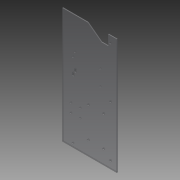
# Autodesk Inventor part: Electrical Board 2
Saved by Autodesk Inventor 2014 SP1 (Build 180222100, 222)
## iProperties
Created: 2013-12-13
Part Number: Electrical Board 2
Material: Polycarbonate, Clear
Document SubType Name: Modeling
Designer: Moses
Mass: 324.91 g
Surface Area: 1758.42 cm^2
Volume: 270.758 cm^3
Density: 1.2 g/cm^3
Appearance: Polycarbonate - Clear
Author: Moses
Autodesk Inventor part; units mm, degrees
ref_plane "YZ Plane" through (0, 0, 0) normal (1, 0, 0) x (0, 1, 0)
ref_plane "XZ Plane" through (0, 0, 0) normal (0, 1, 0) x (-1, 0, 0)
ref_plane "XY Plane" through (0, 0, 0) normal (0, 0, 1) x (1, 0, 0)
sketch "Sketch1" plane through (0, 0, 0) normal (0, 0, 1) x (1, 0, 0)
  line L0 (0, 0) -> (203.2, 0)
  line L1 (203.2, 0) -> (203.2, 431.8)
  line L2 (203.2, 431.8) -> (170.815, 431.8)
  line L3 (0, 431.8) -> (0, 0)
  circle A0 centre (177.8, 406.4) radius 3.3782
  circle A1 centre (177.8, 215.9) radius 3.3782
  circle A2 centre (177.8, 25.4) radius 3.3782
  line L4 (203.2, 215.9) -> (0, 215.9) construction
  line L5 (94.615, 431.8) -> (145.415, 393.7)
  line L6 (145.415, 393.7) -> (170.815, 393.7)
  line L7 (170.815, 393.7) -> (170.815, 431.8)
  line L8 (94.615, 431.8) -> (0, 431.8)
  line L9 (170.815, 431.8) -> (94.615, 431.8)
  circle A3 centre (139.7, 304.8) radius 2.3495
  line L10 (139.7, 304.8) -> (139.7, 246.634) construction
  circle A4 centre (139.7, 246.634) radius 2.3495
  circle A5 centre (45.6, 310.6) radius 2.54
  circle A6 centre (38.1, 292.1) radius 2.54
  line L11 (45.6, 310.6) -> (38.1, 310.6) construction
  line L12 (38.1, 310.6) -> (38.1, 292.1) construction
  line L13 (38.1, 292.1) -> (45.6, 292.1) construction
  line L14 (45.6, 292.1) -> (45.6, 310.6) construction
  circle A7 centre (38.1, 12.7) radius 2.3495
  line L15 (71.1544, 389.1684) -> (109.2544, 389.1684) construction
  line L16 (109.2544, 389.1684) -> (109.2544, 370.1184) construction
  line L17 (109.2544, 370.1184) -> (71.1544, 370.1184) construction
  line L18 (71.1544, 370.1184) -> (71.1544, 389.1684) construction
  line L19 (95.25, 165.1) -> (152.4, 165.1) construction
  line L20 (152.4, 165.1) -> (152.4, 50.8) construction
  line L21 (152.4, 50.8) -> (95.25, 50.8) construction
  line L22 (95.25, 50.8) -> (95.25, 165.1) construction
  circle A8 centre (95.25, 165.1) radius 3.175
  circle A9 centre (152.4, 165.1) radius 3.175
  circle A10 centre (152.4, 50.8) radius 3.175
  circle A11 centre (95.25, 50.8) radius 3.175
  line L23 (30.6, 229.55) -> (30.6, 259.55) projected
  arc A12 (30.6, 229.55) -> (34.6, 225.55) centre (34.6, 229.55) ccw projected
  line L24 (52.6, 225.55) -> (34.6, 225.55) projected
  line L25 (52.6, 225.55) -> (52.6, 263.55) projected
  line L26 (34.6, 263.55) -> (52.6, 263.55) projected
  arc A13 (34.6, 263.55) -> (30.6, 259.55) centre (34.6, 259.55) ccw projected
  arc A14 (49.81, 256.2) -> (44.31, 256.2) centre (47.06, 256.2) ccw projected
  line L27 (49.81, 256.2) -> (49.81, 248.7) projected
  arc A15 (44.31, 248.7) -> (49.81, 248.7) centre (47.06, 248.7) ccw projected
  line L28 (44.31, 248.7) -> (44.31, 256.2) projected
  arc A16 (41.85, 240.2) -> (36.35, 240.2) centre (39.1, 240.2) ccw projected
  line L29 (41.85, 240.2) -> (41.85, 232.7) projected
  arc A17 (36.35, 232.7) -> (41.85, 232.7) centre (39.1, 232.7) ccw projected
  line L30 (36.35, 232.7) -> (36.35, 240.2) projected
  circle A18 centre (30.4488, 139.597) radius 2.3812 projected
  circle A19 centre (64.8012, 139.597) radius 2.3812 projected
  circle A20 centre (30.4488, 106.323) radius 2.3812 projected
  circle A21 centre (64.8012, 106.323) radius 2.3812 projected
  dimension "d0" = 6.7564
  dimension "d3" = 190.5
  dimension "d8" = 25.4
  dimension "d9" = 431.8
  dimension "d10" = 203.2
  dimension "d14" = 38.1
  dimension "d15" = 76.2
  dimension "d16" = 25.4
  dimension "d17" = 4.699
  dimension "d18" = 58.166
  dimension "d19" = 63.5
  dimension "d20" = 127
  dimension "d26" = 5.08
  dimension "d27" = 18.5
  dimension "d28" = 7.5
  dimension "d29" = 38.1
  dimension "d30" = 76.2
  dimension "d31" = 4.699
  dimension "d32" = 38.1
  dimension "d33" = 12.7
  dimension "d34" = 32.385
  dimension "d35" = 19.05
  dimension "d36" = 38.1
  dimension "d37" = 57.15
  dimension "d38" = 6.35
  dimension "d39" = 114.3
  dimension "d40" = 50.8
  dimension "d41" = 50.8
  constraints: 46 end point, 12 centre point, 10 parallel, 5 coincident, 5 equal radius, 5 horizontal, 4 perpendicular, 3 vertical, 2 midpoint, 1 point on line, 4 other
  measures "d0" diameter of A0
  measures "d3" distance of A0.centre A1.centre
  measures "d8" distance from line of L1 A0.centre
  measures "d9" distance of L3.start L0.start
  measures "d10" distance of L0.start L0.end
  measures "d14" distance of L6.end L2.end
  measures "d15" distance of L2.end L5.start
  measures "d16" distance of L5.end L6.end
  measures "d17" diameter of A3
  measures "d18" distance of L10.start L10.end
  measures "d19" distance between parallel lines of L1 L10
  measures "d20" distance from line of L9 L10.start
  measures "d26" diameter of A5
  measures "d27" distance of L14.start L14.end
  measures "d28" distance of L12.end L14.start
  measures "d29" distance between parallel lines of L3 L12
  measures "d30" distance between parallel lines of L4 L13
  measures "d31" diameter of A7
  measures "d32" distance from line of A7.centre L3
  measures "d33" distance from line of L0 A7.centre
  measures "d34" distance between parallel lines of L1 L7
  measures "d35" distance of L15.end L16.end
  measures "d36" distance of L16.end L17.end
  measures "d37" distance of L19.start L19.end
  measures "d38" diameter of A8
  measures "d39" distance of L21.end L19.start
  measures "d40" distance between parallel lines of L0 L21
  measures "d41" distance between parallel lines of L1 L20
extrude "Extrusion1" add sketch "Sketch1" along normal blind 3.175 contours L3 L8 L5 L6 L7 L2 L1 L0 | L23 A13 L26 L25 L24 A12
body "Solid1"
